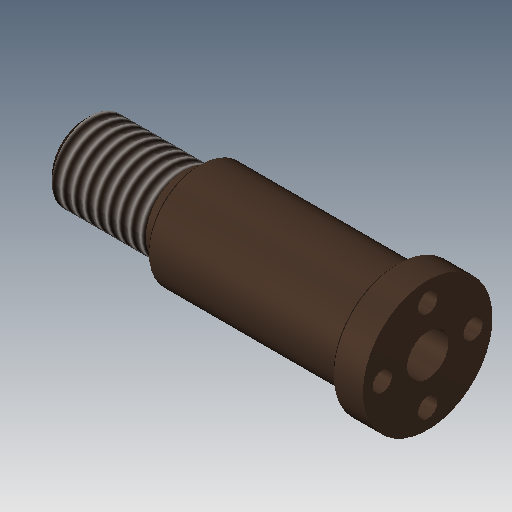
# Autodesk Inventor part: BronzeHollowScrew
Saved by Autodesk Inventor 2019.4 (Build 234330000, 330)
## iProperties
Created: 2020-02-28
Part Number: BronzeHollowScrew
Material: Bronze, Soft Tin
Document SubType Name: Modeling
Designer: Peter
Mass: 69.5524 g
Surface Area: 42.2782 cm^2
Volume: 7.84131 cm^3
Density: 8.874 g/cm^3
Appearance: Bronze - Satin
Author: Peter
Autodesk Inventor part; units mm, degrees
ref_plane "YZ Plane" through (0, 0, 0) normal (1, 0, 0) x (0, 1, 0)
ref_plane "XZ Plane" through (0, 0, 0) normal (0, 1, 0) x (-1, 0, 0)
ref_plane "XY Plane" through (0, 0, 0) normal (0, 0, 1) x (1, 0, 0)
sketch "Sketch1" plane through (0, 0, 0) normal (0, 0, 1) x (1, 0, 0)
  line L0 (0, 0) -> (0, 10)
  line L1 (0, 10) -> (-5, 10)
  line L2 (-5, 10) -> (-5, 8)
  line L3 (-5, 8) -> (-35.5, 8)
  line L4 (-35.5, 8) -> (-35.5, 6)
  line L5 (-35.5, 6) -> (-53, 6)
  line L6 (-53, 6) -> (-53, 0)
  line L7 (-53, 0) -> (0, 0)
  dimension "d1" = 10
  dimension "d2" = 5
  dimension "d3" = 2
  dimension "d4" = 2
  dimension "d5" = 35.5
  dimension "d6" = 53
  constraints: 16 end point, 6 perpendicular, 1 horizontal, 1 vertical
  measures "d1" distance of L0.start L0.end
  measures "d2" distance of L0.end L1.end
  measures "d3" distance of L1.end L2.end
  measures "d4" distance of L3.end L4.end
  measures "d5" distance between parallel lines of L0 L4
  measures "d6" distance between parallel lines of L0 L6
revolve "Revolution1" add sketch "Sketch1" angle 360 about axis through (-53, 0, 0) along (1, 0, 0)
thread "Thread1" size "M12x1.75" class "6g" standard "ISO Metric profile" length 16 offset 2
chamfer "Chamfer1" distance 1 angle 45 1 edges at (-53, -6, 0)
chamfer "Chamfer2" distance 0.5 angle 45 2 edges at (-35.5, -8, 0) (-5, -10, 0)
sketch "Sketch2" plane through (0, 0, 0) normal (1, 0, 0) x (0, 0, -1)
  circle A0 centre (0, 0) radius 7
  dimension "d17" = 14
  constraints: 1 centre point, 1 coincident
  measures "d17" diameter of A0
hole "Hole1" at (0, 0, 0) direction (-1, 0, 0) diameter 6.35 end through all
sketch "Sketch3" plane through (0, 0, 0) normal (1, 0, 0) x (0, 0, -1)
  circle A0 centre (0, 0) radius 7
  line L0 (0, 0) -> (-7, 0)
  dimension "d25" = 14
  constraints: 2 end point, 1 coincident, 1 horizontal, 1 horizontal alignment, 2 other
hole "Hole2" at (0, 0, 7) direction (-1, 0, 0) diameter 3 depth 4.5 tip angle 118
pattern_circular "Circular Pattern1" count 4 over 360 about axis through (-60.075, 0, 0) along (1, 0, 0) of "Hole2"
body "Solid1"
